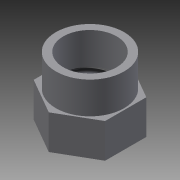
# Autodesk Inventor part: HexCap
Saved by Autodesk Inventor 2015 (Build 190159000, 159)
## iProperties
Created: 2016-02-20
Part Number: HexCap
Material: Generic
Document SubType Name: Modeling
Designer: Owner
Density: 1 g/cm^3
Appearance: Default
Author: Owner
Autodesk Inventor part; units mm, degrees
ref_plane "YZ Plane" through (0, 0, 0) normal (1, 0, 0) x (0, 1, 0)
ref_plane "XZ Plane" through (0, 0, 0) normal (0, 1, 0) x (-1, 0, 0)
ref_plane "XY Plane" through (0, 0, 0) normal (0, 0, 1) x (1, 0, 0)
sketch "Sketch1" plane through (0, 0, 0) normal (0, 1, 0) x (-1, 0, 0)
  line L0 (0, 0) -> (3.5635, -2.0574)
  line L1 (0, 0) -> (4.1148, 0) construction
  line L2 (3.5635, -2.0574) -> (3.5635, -6.1722)
  line L3 (3.5635, -6.1722) -> (0, -8.2296)
  line L4 (0, -8.2296) -> (-3.5635, -6.1722)
  line L5 (-3.5635, -6.1722) -> (-3.5635, -2.0574)
  line L6 (-3.5635, -2.0574) -> (0, 0)
  dimension "d0" = 4.1148
  dimension "d1" = 30
  dimension "d2" = 4.1148
  dimension "d3" = 4.1148
  dimension "d4" = 120
  constraints: 14 end point, 2 parallel, 1 equal length, 1 horizontal, 1 vertical
  measures "d0" distance of L0.start L0.end
  measures "d1" angle of L0 L1
  measures "d2" distance of L0.end L2.end
  measures "d3" distance of L2.end L3.end
  measures "d4" angle of L2 L3
extrude "Extrusion1" add sketch "Sketch1" along normal blind 3.429
sketch "Sketch2" plane through (0, 3.429, 0) normal (0, 1, 0) x (1, 0, 0)
  line L0 (-3.5635, 2.0574) -> (0, 0) projected
  line L1 (0, 0) -> (3.5635, 2.0574) projected
  line L2 (3.5635, 2.0574) -> (3.5635, 6.1722) projected
  line L3 (3.5635, 6.1722) -> (0, 8.2296) projected
  line L4 (0, 8.2296) -> (-3.5635, 6.1722) projected
  line L5 (-3.5635, 6.1722) -> (-3.5635, 2.0574) projected
  line L6 (0, 0) -> (0, 4.1148) construction
  circle A0 centre (0, 4.1148) radius 3.4036
  dimension "d8" = 6.8072
  constraints: 2 end point, 1 centre point, 1 coincident, 1 vertical
  measures "d8" diameter of A0
extrude "Extrusion2" add sketch "Sketch2" along normal blind 3.175 contours A0
hole "Hole1" at (0, 6.604, -4.1148) direction (0, -1, 0) diameter 5.334 end through all
thread "Thread1" size "12-24 UNC" class "2B" standard "ANSI Unified Screw Threads" length 3.429
body "Solid1"
